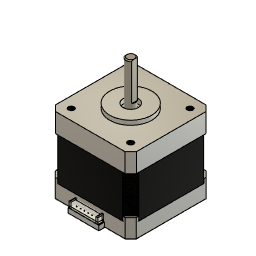
DIY-Camera-Slider-2020 v37 (Autodesk Fusion 360 archive; units mm, degrees)
design "STEPPER MOTOR NEMA 17"
Autodesk Fusion 360 part; units mm, degrees
sketch "Sketch2" plane through (0, 0, 0) normal (0, 1, 0) x (1, 0, 0)
  line L0 (21.15, 21.15) -> (-21.15, 21.15)
  line L1 (-21.15, 21.15) -> (-21.15, -21.15)
  line L2 (-21.15, -21.15) -> (21.15, -21.15)
  line L3 (21.15, -21.15) -> (21.15, 21.15)
  line L4 (21.15, 21.15) -> (-21.15, -21.15) construction
  line L5 (-21.15, 21.15) -> (21.15, -21.15) construction
  dimension "d3" = 42.3
  dimension "d4" = 42.3
  constraint horizontal L0
  constraint perpendicular L0 L1
  constraint parallel L0 L2
  constraint parallel L1 L3
  constraint coincident L4 origin
  constraint coincident L5 origin
  measures "d3" distance of L1.end L2.end
  measures "d4" distance of L0.end L1.end
extrude "Extrude1" add sketch "Sketch2" along normal blind 10 makes body 1
chamfer "Chamfer1" distance 2.9 angle 45 4 edges at (-21.15, 5, 21.15) (21.15, 5, 21.15) (21.15, 5, -21.15) (-21.15, 5, -21.15) on bodies 1
sketch "Sketch3" plane through (0, 0, 0) normal (0, 0, 1) x (1, 0, 0)
  line L0 (22.4607, 12.2, -17.092) -> (22.4607, 12.2, 16.935)
  line L1 (22.4607, 7.8, -17.092) -> (22.4607, 12.2, -17.092)
  line L2 (22.4607, 12.2, 16.935) -> (22.4607, 7.8, -17.092) construction
  line L3 (22.4607, 7.8, 16.935) -> (22.4607, 7.8, -17.092)
  line L4 (22.4607, 12.2, 16.935) -> (22.4607, 7.8, 16.935)
  dimension "d9" = 4.4
extrude "Extrude2" cut sketch "Sketch3" against normal blind 50 contours L0 L1 L3 L4 in plane through (22.4607, 0, 0) normal (1, 0, 0) bodies 1
sketch "Sketch4" plane through (0, 0, 0) normal (0, 0, 1) x (1, 0, 0)
  line L0 (-16.9547, 12.2, -25) -> (16.9547, 12.2, -25)
  line L1 (16.9547, 12.2, -25) -> (16.9547, 7.8, -25)
  line L2 (16.9547, 7.8, -25) -> (-16.9547, 7.8, -25)
  line L3 (-16.9547, 7.8, -25) -> (-16.9547, 12.2, -25)
  line L4 (-16.9547, 12.2, -25) -> (16.9547, 7.8, -25) construction
  line L5 (16.9547, 12.2, -25) -> (-16.9547, 7.8, -25) construction
  point P0 (0, 10)
  dimension "d13" = 4.4
extrude "Extrude3" cut sketch "Sketch4" along normal blind 50 contours L0 L1 L2 L3 in plane through (0, 0, -25) normal (0, 0, 1) bodies 1
sketch "Sketch5" plane through (0, 0, 0) normal (0, 0, 1) x (1, 0, 0)
sketch "Sketch6" plane through (0, 7.8, 0) normal (0, 1, 0) x (-1, 0, 0)
  line L0 (16.9547, -17.092) -> (21.15, -17.092)
  line L1 (21.15, -17.092) -> (21.15, 16.935)
  line L2 (21.15, 16.935) -> (16.9547, 16.935)
  line L3 (16.9547, 16.935) -> (16.9547, 21.15)
  line L4 (16.9547, 21.15) -> (-16.9547, 21.15)
  line L5 (-16.9547, 21.15) -> (-16.9547, 16.935)
  line L6 (-16.9547, 16.935) -> (-21.15, 16.935)
  line L7 (-21.15, 16.935) -> (-21.15, -17.092)
  line L8 (-21.15, -17.092) -> (-16.9547, -17.092)
  line L9 (-16.9547, -17.092) -> (-16.9547, -21.15)
  line L10 (-16.9547, -21.15) -> (16.9547, -21.15)
  line L11 (16.9547, -21.15) -> (16.9547, -17.092)
  line L12 (-21.15, 21.15) -> (21.15, 21.15)
  line L13 (21.15, 21.15) -> (21.15, -21.15)
  line L14 (21.15, -21.15) -> (-21.15, -21.15)
  line L15 (-21.15, -21.15) -> (-21.15, 21.15)
  line L16 (-21.15, 21.15) -> (21.15, -21.15) construction
  line L17 (21.15, 21.15) -> (-21.15, -21.15) construction
  dimension "d16" = 42.3
  dimension "d17" = 42.3
  constraint horizontal L12
  constraint perpendicular L12 L13
  constraint parallel L12 L14
  constraint parallel L13 L15
  constraint coincident L16 origin
  constraint coincident L17 origin
  measures "d16" distance of L12.end L13.end
  measures "d17" distance of L12.start L12.end
extrude "Extrude4" add sketch "Sketch6" along normal blind 22 separate body makes body 2
chamfer "Chamfer2" distance 4.2 angle 45 4 edges at (-21.15, 18.8, -21.15) (-21.15, 18.8, 21.15) (21.15, 18.8, -21.15) (21.15, 18.8, 21.15) on bodies 2
sketch "Sketch7" plane through (0, 29.8, 0) normal (0, 1, 0) x (-1, 0, 0)
  line L0 (-16.95, 21.15) -> (-21.15, 16.95)
  line L1 (-21.15, 16.95) -> (-21.15, -16.95)
  line L2 (-21.15, -16.95) -> (-16.95, -21.15)
  line L3 (-16.95, -21.15) -> (16.95, -21.15)
  line L4 (16.95, -21.15) -> (21.15, -16.95)
  line L5 (21.15, -16.95) -> (21.15, 16.95)
  line L6 (21.15, 16.95) -> (16.95, 21.15)
  line L7 (16.95, 21.15) -> (-16.95, 21.15)
  line L8 (-21.15, 21.15) -> (21.15, 21.15)
  line L9 (21.15, 21.15) -> (21.15, -21.15)
  line L10 (21.15, -21.15) -> (-21.15, -21.15)
  line L11 (-21.15, -21.15) -> (-21.15, 21.15)
  line L12 (-21.15, 21.15) -> (21.15, -21.15) construction
  line L13 (21.15, 21.15) -> (-21.15, -21.15) construction
  dimension "d21" = 42.3
  constraint horizontal L8
  constraint perpendicular L8 L9
  constraint parallel L8 L10
  constraint parallel L9 L11
  constraint coincident L12 origin
  constraint coincident L13 origin
  measures "d21" distance of L8.end L9.end
move_body "Move1" bodies 1 2 to x (1, 0, 0) y (0, 1, 0) z (0, 0, 1) at (0, -10, 0)
move_body "Move2" bodies 1 2 to x (1, 0, 0) y (0, 1, 0) z (0, 0, 1) at (0, -10, 0)
extrude "Extrude5" add sketch "Sketch7" along normal blind 10 separate body makes body 3
chamfer "Chamfer3" distance 3 angle 45 4 edges at (-21.15, 34.8, -21.15) (-21.15, 34.8, 21.15) (21.15, 34.8, 21.15) (21.15, 34.8, -21.15) on bodies 3
move_body "Move3" bodies 2 1 to x (1, 0, 0) y (0, 1, 0) z (0, 0, 1) at (0, 20, 0)
sketch "Sketch8" plane through (0, 39.8, 0) normal (0, 1, 0) x (-1, 0, 0)
  line L0 (-21.15, -18.15) -> (-18.15, -21.15)
  line L1 (-18.15, -21.15) -> (18.15, -21.15)
  line L2 (18.15, -21.15) -> (21.15, -18.15)
  line L3 (21.15, -18.15) -> (21.15, 18.15)
  line L4 (21.15, 18.15) -> (18.15, 21.15)
  line L5 (18.15, 21.15) -> (-18.15, 21.15)
  line L6 (-18.15, 21.15) -> (-21.15, 18.15)
  line L7 (-21.15, 18.15) -> (-21.15, -18.15)
  circle A0 centre (0, 0) radius 10.95
  dimension "d26" = 21.9
  constraint coincident A0.centre origin
  measures "d26" diameter of A0
extrude "Extrude6" add sketch "Sketch8" along normal blind 2.3 contours A0 bodies 3
sketch "Sketch9" plane through (0, 42.1, 0) normal (0, 1, 0) x (-1, 0, 0)
  circle A0 centre (0, 0) radius 10.95
  circle A1 centre (0, 0) radius 4
  dimension "d29" = 8
  constraint concentric A0 A1
  measures "d29" diameter of A1
extrude "Extrude7" cut sketch "Sketch9" against normal blind 2.5 contours A1 bodies 3
sketch "Sketch10" plane through (0, 0, 0) normal (0, 1, 0) x (1, 0, 0)
  circle A0 centre (0, 0) radius 4.6
  dimension "d32" = 9.2
  constraint coincident A0.centre origin
  measures "d32" diameter of A0
extrude "Extrude8" cut sketch "Sketch10" along normal blind 3.4 bodies 1
sketch "Sketch11" plane through (0, 42.1, 0) normal (0, 1, 0) x (-1, 0, 0)
  circle A0 centre (0, 0) radius 4
  circle A1 centre (0, 0) radius 10.95
  circle A2 centre (0, 0) radius 2.5
  dimension "d35" = 5
  constraint coincident A0.centre A1.centre
  measures "d35" diameter of A2
extrude "Extrude9" add sketch "Sketch11" along normal blind 61 separate body contours A2 makes body 4
move_body "Move4" bodies 4 to x (1, 0, 0) y (0, 1, 0) z (0, 0, 1) at (0, -40, 0)
sketch "Sketch12" plane through (0, 39.6, 0) normal (0, 1, 0) x (-1, 0, 0)
  circle A0 centre (0, 0) radius 4
  line L0 (-2.5, -2.5, 4) -> (-2, -2.5, 4)
  line L1 (-2, -2.5, 4) -> (-2, 2, 4)
  line L2 (-2, 2, 4) -> (-2.5, 2, 4)
  line L3 (-2.5, 2, 4) -> (-2.5, -2.5, 4)
sketch "Sketch13" plane through (2.25, 43.6, -0.25) normal (0, 1, 0) x (-1, 0, 0)
fillet "Fillet1" radius 0.5 1 edges at (2.3308, 63.1, -0.904) on bodies 4
extrude "Extrude10" cut sketch "Sketch12" along normal blind 22 contours L0 L1 L2 L3 in plane through (0, 43.6, 0) normal (0, 1, 0) bodies 4
fillet "Fillet2" radius 0.4 8 edges at (-21.15, 0, 0) (0, 0, -21.15) (-19.7, 0, -19.7) (-19.7, 0, 19.7) (0, 0, 21.15) (19.7, 0, 19.7) (21.15, 0, 0) (19.7, 0, -19.7) on bodies 1
sketch "Sketch15" plane through (2.25, 43.6, -0.25) normal (0, 1, 0) x (-1, 0, 0)
sketch "Sketch16" plane through (0, 0, 0) normal (0, 0, 1) x (1, 0, 0)
sketch "Sketch17" plane through (0, 42.1, 0) normal (0, 1, 0) x (-1, 0, 0)
  circle A0 centre (0, 0) radius 4
  circle A1 centre (0, 0) radius 10.95
  circle A2 centre (0, 0) radius 2.75
  dimension "d45" = 5.5
  constraint concentric A0 A2
  measures "d45" diameter of A2
extrude "Extrude11" cut sketch "Sketch17" against normal blind 55 contours A2 bodies 1 2 3
copy_body "Body->Comp1" bodies 1 removing the originals makes body 5 in component "Component"
copy_body "Body->Comp2" bodies 3 removing the originals makes body 6 in component "Component'"
copy_body "Body->Comp3" bodies 4 removing the originals makes body 7 in component "Component''"
copy_body "Body->Comp4" bodies 2 removing the originals makes body 8 in component "Component'''"
sketch "Sketch18" plane through (0, 0, 0) normal (0, 1, 0) x (1, 0, 0)
  circle A0 through (-14, 15.5, 40) (-16.25, 16.799, 40) (-16.25, 14.201, 40)
  circle A1 through (-14, -15.5, 40) (-16.25, -14.201, 40) (-16.25, -16.799, 40)
  circle A2 through (17, 15.5, 40) (14.75, 16.799, 40) (14.75, 14.201, 40)
  circle A3 through (17, -15.5, 40) (14.75, -14.201, 40) (14.75, -16.799, 40)
  dimension "d52" = 3
  dimension "d53" = 3
  dimension "d54" = 31
  dimension "d58" = 3
  dimension "d59" = 3
  dimension "d87" = 31
  dimension "d88" = 31
extrude "Extrude1'" cut sketch "Sketch18" against normal blind 5 contours A0 | A1 | A2 | A3 in plane through (0, 40, 0) normal (0, 1, 0) bodies 6 in component "Component'"
thread "Thread1" "ISO Metric profile 3.0 M3x0.5 6H" major diameter 3.086 minor diameter 2.529 pitch 0.5 angle 60 resizes the face on face at (-14.0075, 38.2, -15.3506) on bodies 6 in component "Component'"
thread "Thread2" "ISO Metric profile 3.0 M3x0.5 6H" major diameter 3.086 minor diameter 2.529 pitch 0.5 angle 60 resizes the face on face at (-14.0075, 38.2, 15.6494) on bodies 6 in component "Component'"
thread "Thread3" "ISO Metric profile 3.0 M3x0.5 6H" major diameter 3.086 minor diameter 2.529 pitch 0.5 angle 60 resizes the face on face at (16.9925, 38.2, -15.3506) on bodies 6 in component "Component'"
thread "Thread4" "ISO Metric profile 3.0 M3x0.5 6H" major diameter 3.086 minor diameter 2.529 pitch 0.5 angle 60 resizes the face on face at (16.9925, 38.2, 15.6494) on bodies 6 in component "Component'"
sketch "Sketch19" plane through (0, 42.1, 0) normal (0, 1, 0) x (-1, 0, 0)
  circle A0 centre (0, 0) radius 4
  circle A1 centre (0, 0) radius 10.95
  line L0 (-7.3165, 24.4923) -> (8.6835, 24.4923)
  line L1 (8.6835, 24.4923) -> (8.6835, 21.4923)
  line L2 (8.6835, 21.4923) -> (-7.3165, 21.4923)
  line L3 (-7.3165, 21.4923) -> (-7.3165, 24.4923)
  line L4 (-7.3165, 24.4923) -> (8.6835, 21.4923) construction
  line L5 (8.6835, 24.4923) -> (-7.3165, 21.4923) construction
  point P0 (0.6835, 22.9923)
  dimension "d63" = 3
  constraint horizontal L0
  constraint perpendicular L0 L1
  constraint parallel L0 L2
  constraint parallel L1 L3
  constraint coincident L4 P0
  constraint coincident L5 P0
  measures "d63" distance of L0.end L1.end
extrude "Extrude12" add sketch "Sketch19" along normal blind 2.5 separate body contours L0 L1 L2 L3 makes body 9
move_body "Move5" bodies 9 to x (1, 0, 0) y (0, 1, 0) z (0, 0, 1) at (0, -42, -0.5)
move_body "Move6" bodies 9 to x (1, 0, 0) y (0, 1, 0) z (0, 0, 1) at (0, -0.1, 0)
sketch "Sketch20" plane through (0, 42.1, 0) normal (0, 1, 0) x (-1, 0, 0)
  circle A0 centre (0, 0) radius 4
  circle A1 centre (0, 0) radius 10.95
  line L0 (8.1835, 22, -39.6) -> (8.1835, 25, -39.6)
  line L1 (8.1835, 25, -39.6) -> (7.1835, 25, -39.6)
  line L2 (7.1835, 25, -39.6) -> (7.1835, 22, -39.6)
  line L3 (7.1835, 22, -39.6) -> (8.1835, 22, -39.6)
  line L4 (-6.8165, 25, -39.6) -> (-5.8165, 25, -39.6)
  line L5 (-5.8165, 25, -39.6) -> (-5.8165, 22, -39.6)
  line L6 (-5.8165, 22, -39.6) -> (-6.8165, 22, -39.6)
  line L7 (-6.8165, 22, -39.6) -> (-6.8165, 25, -39.6)
  point P0 (8.6835, 23.9923)
  point P1 (-7.3165, 23.9923)
  dimension "d66" = 1
extrude "Extrude13" add sketch "Sketch20" along normal blind 5 separate body contours L0 L1 L2 L3 | L4 L5 L6 L7 in plane through (0, 2.5, 0) normal (0, 1, 0) makes body 10 at (-7.1835, 4.1667, 24) makes body 11 at (5.8165, 4.1667, 24)
move_body "Move7" bodies 10 11 to x (1, 0, 0) y (0, 1, 0) z (0, 0, 1) at (0, 0, -1)
sketch "Sketch21" plane through (0, 42.1, 0) normal (0, 1, 0) x (-1, 0, 0)
  circle A0 centre (0, 0) radius 4
  circle A1 centre (0, 0) radius 10.95
  line L0 (8.1, 25.7, -39.6) -> (-6.75, 25.7, -39.6)
  line L1 (-6.75, 25.7, -39.6) -> (-6.75, 28.4, -39.6)
  line L2 (-6.75, 28.4, -39.6) -> (8.1, 28.4, -39.6)
  line L3 (8.1, 28.4, -39.6) -> (8.1, 25.7, -39.6)
extrude "Extrude14" add sketch "Sketch21" along normal blind 1 separate body contours L0 L1 L2 L3 in plane through (0, 2.5, 0) normal (0, 1, 0) makes body 12
move_body "Move8" bodies 12 to x (1, 0, 0) y (0, 1, 0) z (0, 0, 1) at (0, 0, -4.5)
move_face "MoveFace1" by (0, -1.5, 0) 2 faces at (-7.8501, 7.5, 22) (6.1499, 7.5, 22) on bodies 10 11
sketch "Sketch22" plane through (0, 0, 23.9) normal (0, 0, 1) x (1, 0, 0)
  line L0 (-8.1, 2.5) -> (6.75, 2.5)
  line L1 (6.75, 2.5) -> (6.75, 3.5)
  line L2 (6.75, 3.5) -> (-8.1, 3.5)
  line L3 (-8.1, 3.5) -> (-8.1, 2.5)
  circle A0 centre (-4.5, 5) radius 0.25
  circle A1 centre (-2.5, 5) radius 0.25
  circle A2 centre (-0.5, 5) radius 0.25
  circle A3 centre (1.5, 5) radius 0.25
  circle A4 centre (3.5, 5) radius 0.25
  dimension "d73" = 0.5
  dimension "d74" = 0.5
  dimension "d75" = 0.5
  dimension "d76" = 0.5
  dimension "d77" = 0.5
  measures "d73" diameter of A0
  measures "d74" diameter of A1
  measures "d75" diameter of A2
  measures "d76" diameter of A3
  measures "d77" diameter of A4
extrude "Extrude15" add sketch "Sketch22" against normal blind 2.7 separate body contours A0 | A1 | A2 | A3 | A4 makes body 13 at (-0.2503, 4.9875, 22.1) makes body 14 at (-2.2503, 4.9875, 22.1) makes body 15 at (1.7497, 4.9875, 22.1) makes body 16 at (-4.3644, 5.21, 22.1) makes body 17 at (3.7497, 4.9875, 22.1)
move_body "Move9" bodies 17 16 15 14 13 to x (1, 0, 0) y (0, 1, 0) z (0, 0, 1) at (0, 0, -0.05)
move_body "Move10" bodies 17 14 13 16 15 to x (1, 0, 0) y (0, 1, 0) z (0, 0, 1) at (0, 0, -0.05)
chamfer "Chamfer4" distance 0.12 angle 45 5 edges at (3.2669, 4.9096, 23.8) (1.2669, 4.9096, 23.8) (-2.7331, 4.9096, 23.8) (-4.7331, 4.9096, 23.8) (-0.7331, 4.9096, 23.8) on bodies 13 14 15 16 17
fillet "Fillet3" chord length 0.5 tangency weight 1.68369 6 edges at (-8.1835, 6, 22.5) (-7.1835, 6, 22.5) (-7.6835, 6, 24) (6.3165, 6, 24) (5.8165, 6, 22.5) (6.8165, 6, 22.5) on bodies 10 11
copy_body "CopyPasteBodies1" bodies 12 makes body 18
move_body "Move11" bodies 18 to x (1, 0, 0) y (0, 1, 0) z (0, 0, 1) at (0, 0, 0)
move_body "Move12" bodies 18 to x (1, 0, 0) y (0, 0, -1) z (0, 1, 0) at (0, -18.2, 24.2)
copy_body "Body->Comp5" bodies 18 removing the originals makes body 19 in component "Component''''"
copy_body "Body->Comp6" bodies 10 removing the originals makes body 20 in component "Component'''''"
copy_body "Body->Comp7" bodies 11 removing the originals makes body 21 in component "Component''''''"
copy_body "Body->Comp8" bodies 14 removing the originals makes body 22 in component "Component'''''''"
copy_body "Body->Comp9" bodies 13 removing the originals makes body 23 in component "Component''''''''"
copy_body "Body->Comp10" bodies 16 removing the originals makes body 24 in component "Component'''''''''"
copy_body "Body->Comp11" bodies 17 removing the originals makes body 25 in component "Component''''''''''"
copy_body "Body->Comp12" bodies 15 removing the originals makes body 26 in component "Component'''''''''''"
copy_body "Body->Comp13" bodies 9 removing the originals makes body 27 in component "Component''''''''''''"
copy_body "Body->Comp14" bodies 12 removing the originals makes body 28 in component "Component'''''''''''''"
thread "Thread5" "ISO Metric profile 3.0 M3x0.5 6H" major diameter 3.086 minor diameter 2.529 pitch 0.5 angle 60 modelled right hand crest width 0.1368 on face at (16.7582, 38.2, 15.6259) crest through (16.7645, 39.675, 15.5) on bodies 6 in component "Component'"
thread "Thread6" "ISO Metric profile 3.0 M3x0.5 6H" major diameter 3.086 minor diameter 2.529 pitch 0.5 angle 60 modelled right hand crest width 0.1368 on face at (-14.2418, 38.2, 15.6259) crest through (-14.2355, 39.675, 15.5) on bodies 6 in component "Component'"
thread "Thread7" "ISO Metric profile 3.0 M3x0.5 6H" major diameter 3.086 minor diameter 2.529 pitch 0.5 angle 60 modelled right hand crest width 0.1368 on face at (16.7582, 38.2, -15.3741) crest through (16.7645, 39.675, -15.5) on face at (-14.2418, 38.2, -15.3741) crest through (-14.2355, 39.675, -15.5) on bodies 6 in component "Component'"
component "Component" placed x (1, 0, 0) y (0, 1, 0) z (0, 0, 1) at (0, 0, 0)
component "Component'" placed x (1, 0, 0) y (0, 1, 0) z (0, 0, 1) at (0, 0, 0)
component "Component''" placed x (1, 0, 0) y (0, 1, 0) z (0, 0, 1) at (0, 0, 0)
component "Component'''" placed x (1, 0, 0) y (0, 1, 0) z (0, 0, 1) at (0, 0, 0)
component "Component''''" placed x (1, 0, 0) y (0, 1, 0) z (0, 0, 1) at (0, 0, 0)
component "Component'''''" placed x (1, 0, 0) y (0, 1, 0) z (0, 0, 1) at (0, 0, 0)
component "Component''''''" placed x (1, 0, 0) y (0, 1, 0) z (0, 0, 1) at (0, 0, 0)
component "Component'''''''" placed x (1, 0, 0) y (0, 1, 0) z (0, 0, 1) at (0, 0, 0)
component "Component''''''''" placed x (1, 0, 0) y (0, 1, 0) z (0, 0, 1) at (0, 0, 0)
component "Component'''''''''" placed x (1, 0, 0) y (0, 1, 0) z (0, 0, 1) at (0, 0, 0)
component "Component''''''''''" placed x (1, 0, 0) y (0, 1, 0) z (0, 0, 1) at (0, 0, 0)
component "Component'''''''''''" placed x (1, 0, 0) y (0, 1, 0) z (0, 0, 1) at (0, 0, 0)
component "Component''''''''''''" placed x (1, 0, 0) y (0, 1, 0) z (0, 0, 1) at (0, 0, 0)
component "Component'''''''''''''" placed x (1, 0, 0) y (0, 1, 0) z (0, 0, 1) at (0, 0, 0)
